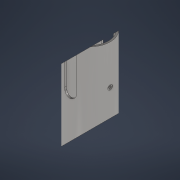
# Autodesk Inventor part: Test_Blade_Guard
Saved by Autodesk Inventor 2022 (Build 260153000, 153)
## iProperties
Created: 2024-05-08
Part Number: Test_Blade_Guard
Material: Generic
Document SubType Name: Modeling
Designer: jo_ki
Density: 1 g/cm^3
Appearance: Steel - Polished
Author: jo_ki
Autodesk Inventor part; units mm, degrees
ref_plane "XZ Plane" through (0, 0, 0) normal (0, 1, 0) x (-1, 0, 0)
ref_plane "XY Plane" through (0, 0, 0) normal (0, 0, 1) x (1, 0, 0)
sketch "Sketch1" plane through (0, 0, 0) normal (0, 0, 1) x (1, 0, 0)
  line L0 (-23.5, -60) -> (23.5, -60)
  line L1 (23.5, -60) -> (23.5, 60)
  line L2 (23.5, 60) -> (-23.5, 60)
  line L3 (-23.5, 60) -> (-23.5, -60)
  line L4 (-23.5, -60) -> (23.5, 60) construction
  line L5 (23.5, -60) -> (-23.5, 60) construction
  line L6 (-23.5, 19.5) -> (17, 60)
  line L7 (-20, -60) -> (23.5, -16.5)
  line L8 (21.5, 60) -> (21.5, -60)
  line L9 (-21.5, 60) -> (-21.5, -60)
  line L10 (0, 60) -> (0, 10.5) construction
  line L11 (-7, 60) -> (-7, 10.5)
  line L12 (7, 10.5) -> (7, 60)
  arc A0 (7, 60) -> (-7, 60) centre (0, 60) ccw
  arc A1 (-7, 10.5) -> (7, 10.5) centre (0, 10.5) ccw
  line L13 (0, 60) -> (0, -60)
  line L14 (0, -85.4) -> (0, 92.4) projected
  point P0 (0, 0)
  point P1 (0, 35.25)
  point P2 (-7, 36)
  point P3 (7, 50)
  dimension "d0" = 2
  dimension "d1" = 2
  dimension "d2" = 47
  dimension "d3" = 14
  dimension "d4" = 120
  dimension "d5" = 56.5
  dimension "d6" = 20
  dimension "d7" = 45
  dimension "d9" = 17
  constraints: 30 end point, 8 point on line, 5 midpoint, 4 parallel, 4 perpendicular, 4 point on circle, 4 tangent, 2 centre point, 1 horizontal
  measures "d0" distance between parallel lines of L1 L8
  measures "d1" distance between parallel lines of L3 L9
  measures "d2" distance between parallel lines of L3 L1
  measures "d3" distance between parallel lines of L11 L12
  measures "d4" distance between parallel lines of L0 L2
  measures "d6" distance from line of L13 L7.start
  measures "d7" angle of L0 L7
  measures "d9" distance from line of L6.end L10
revolve "Revolution1" add sketch "Sketch1" angle 360 about axis through (0, -10, 0) along (0, 1, 0) contours L8 L7 L1 L0 | L8 L2 L1 L7
extrude "Extrusion1" cut sketch "Sketch1" along normal through all both and the other way through all contours L3 L2 L9 L6 | L7 L13 L0 | L9 L2 L11 L6 | L13 L7 L8 L0 | L11 L2 L13 L6 | L6 L13 A1 L11 | L8 L7 L1 L0 | L13 L6 L12 A1 | L13 L2 L12 L6 | A0 L14 L2 | L12 L2 L6 | L14 A0 L2
ref_plane "Work Plane1" through (23.5, 0, 0) normal (1, 0, 0) x (0, 1, 0)
sketch "Sketch2" plane through (23.5, 0, 0) normal (1, 0, 0) x (0, 1, 0)
  arc A0 (60, -16.225) -> (50, 22.4332) centre (43, 0) ccw projected
  line L0 (50, 22.4332) -> (10.5, 22.4332) projected
  line L1 (10.5, 22.4332) -> (36, 22.4332) projected
  arc A1 (36, 22.4332) -> (36, -22.4332) centre (43, 0) ccw projected
  line L2 (36, -22.4332) -> (10.5, -22.4332) projected
  line L3 (10.5, -22.4332) -> (50, -22.4332) projected
  arc A2 (50, -22.4332) -> (60, 16.225) centre (43, 0) ccw projected
  line L4 (60, 16.225) -> (60, -16.225) projected
  arc A3 (-60, -12.339) -> (-60, 12.339) centre (-40, 0) ccw projected
  line L5 (-60, 12.339) -> (-60, -12.339) projected
  line L6 (60, -16.225) -> (60, 16.225) projected
  line L7 (60, 0) -> (-16.5, 0)
  arc A4 (-60, -12.339) -> (-60, 12.339) centre (-40, 0) ccw projected
  point P0 (0, 0)
  point P1 (19.5, 0)
  point P2 (14.5, 0)
  dimension "d20" = 5
  constraints: 3 point on circle, 2 end point, 2 point on line, 1 midpoint
  measures "d20" distance of point (19.5, 0) point (14.5, 0)
hole "Hole1" at (23.5, 14.5, 0) direction (-1, 0, 0) diameter 2.9 depth 5 counterbore diameter 5.5 counterbore depth 0.5 clearance for "Socket Head Cap Screw DIN EN ISO 4762" size "M2.5" standard "DIN"
equation "\"d1\" = d0"
body "Solid1"
